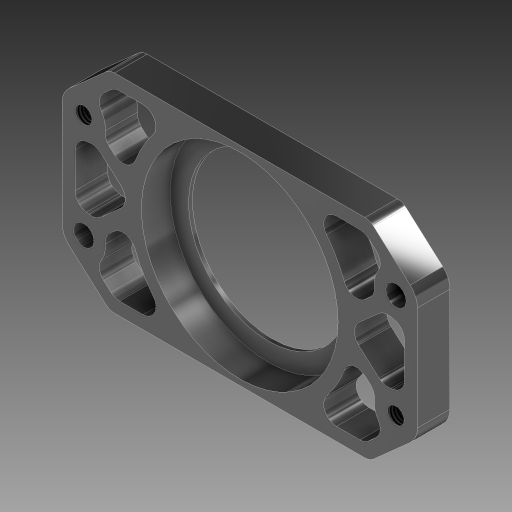
# Autodesk Inventor part: MaxSpline Bearing Block
Saved by Autodesk Inventor 2024 (Build 280153000, 153)
## iProperties
Created: 2023-05-20
Part Number: MaxSpline Bearing Block
Material: Aluminum 6061
Document SubType Name: Modeling
Designer: Max Boord
Mass: 47.5675 g
Surface Area: 134.115 cm^2
Volume: 17.6176 cm^3
Density: 2.7 g/cm^3
Appearance: Glazed - Black
Author: Max Boord
Mass: 32.2811 g
Surface Area: 98.3675 cm^2
Volume: 11.956 cm^3
Appearance: Aluminum - Flat
Autodesk Inventor part; units mm, degrees
ref_plane "YZ Plane" through (0, 0, 0) normal (1, 0, 0) x (0, 1, 0)
ref_plane "XZ Plane" through (0, 0, 0) normal (0, 1, 0) x (-1, 0, 0)
ref_plane "XY Plane" through (0, 0, 0) normal (0, 0, 1) x (1, 0, 0)
sketch "Sketch1" plane through (0, 0, 0) normal (0, 0, 1) x (1, 0, 0)
  circle A0 centre (0, 0) radius 24
  line L0 (31.75, 25.4) -> (-31.75, 25.4)
  line L1 (-31.75, 25.4) -> (-31.75, -25.4)
  line L2 (-31.75, -25.4) -> (31.75, -25.4)
  line L3 (31.75, -25.4) -> (31.75, 25.4)
  line L4 (31.75, 25.4) -> (-31.75, -25.4) construction
  line L5 (-31.75, 25.4) -> (31.75, -25.4) construction
  circle A1 centre (-38.1, 12.7) radius 2.4892 construction
  circle A2 centre (-38.1, -12.7) radius 2.4892
  circle A3 centre (38.1, 12.7) radius 2.4892
  circle A4 centre (38.1, -12.7) radius 2.4892 construction
  arc A5 (-41.6024, 16.6385) -> (-43.3705, 12.7) centre (-38.1, 12.7) ccw
  arc A6 (-43.3705, -12.7) -> (-41.6024, -16.6385) centre (-38.1, -12.7) ccw
  arc A7 (43.3705, 12.7) -> (41.6024, 16.6385) centre (38.1, 12.7) ccw
  arc A8 (41.6024, -16.6385) -> (43.3705, -12.7) centre (38.1, -12.7) ccw
  line L6 (-31.75, 25.4) -> (-41.6024, 16.6385)
  line L7 (-43.3705, 12.7) -> (-43.3705, -12.7)
  line L8 (-41.6024, -16.6385) -> (-31.75, -25.4)
  line L9 (31.75, 25.4) -> (41.6024, 16.6385)
  line L10 (43.3705, 12.7) -> (43.3705, -12.7)
  line L11 (41.6024, -16.6385) -> (31.75, -25.4)
  line L12 (-38.1, 12.7) -> (0, 0) construction
  line L13 (-38.1, -12.7) -> (0, 0) construction
  circle A9 centre (0, 0) radius 19.5
  circle A10 centre (-38.1, 12.7) radius 2.0193
  circle A11 centre (38.1, -12.7) radius 2.0193
  dimension "d0" = 48
  dimension "d1" = 50.8
  dimension "d2" = 4.9784
  dimension "d5" = 25.4
  dimension "d8" = 76.2
  dimension "d11" = 10.541
  dimension "d13" = 6.35
  dimension "d17" = 39
  dimension "d22" = 4.0386
  constraints: 28 end point, 12 centre point, 8 point on circle, 8 tangent, 4 equal radius, 2 coincident, 2 equal length, 2 horizontal, 2 midpoint, 2 parallel, 1 perpendicular, 1 vertical, 6 other
  measures "d0" diameter of A0
  measures "d1" distance of L1.end L0.end
  measures "d2" diameter of A1
  measures "d5" distance of L12.start L13.start
  measures "d8" distance of L12.start A3.centre
  measures "d11" diameter of A6
  measures "d13" distance from line of L1 L12.start
  measures "d17" diameter of A9
  measures "d22" diameter of A10
extrude "Extrusion1" add sketch "Sketch1" along normal blind 7 and the other way blind 0.9375 contours L3 L2 L1 L0 | L9 A7 L10 A8 L11 L3 | L1 L8 A6 L7 A5 L6
extrude "Extrusion2" add sketch "Sketch1" against normal up to surface (0.9375 mm away) contours A0
sketch "Sketch5" plane through (0, 0, 0) normal (0, 1, 0) x (-1, 0, 0)
  line L0 (-6.8199, 0) -> (-6.8199, 10.2616)
  line L1 (-24.003, 10.2616) -> (-24.003, 0)
  line L2 (-24.003, 0) -> (-6.8199, 10.2616) construction
  line L3 (-6.8199, 0) -> (-24.003, 10.2616) construction
  line L4 (-17.6085, 0) -> (-17.6085, 0.3048)
  line L5 (-17.6085, 0.3048) -> (-13.2143, 0.3048)
  line L6 (-13.2143, 0.3048) -> (-13.2143, 0)
  line L7 (-17.6086, 10.2616) -> (-17.6086, 9.9568)
  line L8 (-17.6086, 9.9568) -> (-13.2143, 9.9568)
  line L9 (-13.2143, 9.9568) -> (-13.2143, 10.2616)
  line L10 (-6.8199, 10.2616) -> (-13.2143, 10.2616)
  line L11 (-17.6086, 10.2616) -> (-24.003, 10.2616)
  line L12 (-24.003, 0) -> (-17.6085, 0)
  line L13 (-13.2143, 0) -> (-6.8199, 0)
  line L14 (0, 0) -> (0, -7.8157)
  line L15 (-24, 0) -> (24, 0) projected
  point P0 (-15.4115, 5.1308)
  dimension "d89" = 10.2616
  dimension "d90" = 13.6398
  dimension "d91" = 4.3942
  dimension "d92" = 0.3048
  dimension "d93" = 48.006
  constraints: 30 end point, 7 parallel, 6 equal length, 3 horizontal, 3 perpendicular, 2 midpoint, 1 collinear, 1 point on line, 1 vertical
  measures "d89" distance between parallel lines of L10 L13
  measures "d90" diameter of L0 L14
  measures "d91" distance of L7.end L8.end
  measures "d92" distance of L8.end L9.end
  measures "d93" diameter of L1 L14
revolve "Revolution1" [suppressed]
chamfer "Chamfer2" [suppressed]
sketch "Sketch2" plane through (0, 0, 7) normal (0, 0, 1) x (1, 0, 0)
  arc A0 (-41.6024, 16.6385) -> (-43.3705, 12.7) centre (-38.1, 12.7) ccw projected
  line L0 (-43.3705, 12.7) -> (-43.3705, -12.7) projected
  arc A1 (-43.3705, -12.7) -> (-41.6024, -16.6385) centre (-38.1, -12.7) ccw projected
  line L1 (-41.6024, -16.6385) -> (-31.75, -25.4) projected
  line L2 (-31.75, -25.4) -> (31.75, -25.4) projected
  line L3 (31.75, -25.4) -> (41.6024, -16.6385) projected
  arc A2 (41.6024, -16.6385) -> (43.3705, -12.7) centre (38.1, -12.7) ccw projected
  line L4 (43.3705, -12.7) -> (43.3705, 12.7) projected
  arc A3 (43.3705, 12.7) -> (41.6024, 16.6385) centre (38.1, 12.7) ccw projected
  line L5 (41.6024, 16.6385) -> (31.75, 25.4) projected
  line L6 (31.75, 25.4) -> (-31.75, 25.4) projected
  line L7 (-31.75, 25.4) -> (-41.6024, 16.6385) projected
  circle A4 centre (38.1, -12.7) radius 2.0193 projected
  circle A5 centre (38.1, 12.7) radius 2.4892 projected
  circle A6 centre (0, 0) radius 24 projected
  circle A7 centre (-38.1, -12.7) radius 2.4892 projected
  circle A8 centre (-38.1, 12.7) radius 2.0193 projected
  line L8 (30.5425, -22.225) -> (-30.5425, -22.225)
  line L9 (-30.5425, -22.225) -> (-39.4925, -14.2659)
  arc A9 (-40.1955, -12.7) -> (-39.4925, -14.2659) centre (-38.1, -12.7) ccw
  line L10 (-40.1955, -12.7) -> (-40.1955, 12.7)
  arc A10 (-39.4925, 14.2659) -> (-40.1955, 12.7) centre (-38.1, 12.7) ccw
  line L11 (-39.4925, 14.2659) -> (-30.5425, 22.225)
  line L12 (-30.5425, 22.225) -> (30.5425, 22.225)
  line L13 (30.5425, 22.225) -> (39.4925, 14.2659)
  arc A11 (40.1955, 12.7) -> (39.4925, 14.2659) centre (38.1, 12.7) ccw
  line L14 (40.1955, 12.7) -> (40.1955, -12.7)
  arc A12 (39.4925, -14.2659) -> (40.1955, -12.7) centre (38.1, -12.7) ccw
  line L15 (39.4925, -14.2659) -> (30.5425, -22.225)
  circle A13 centre (0, 0) radius 27.175
  circle A14 centre (38.1, -12.7) radius 5.2705
  circle A15 centre (38.1, 12.7) radius 5.2705
  circle A16 centre (-38.1, 12.7) radius 5.2705
  circle A17 centre (-38.1, -12.7) radius 5.2705
  line L16 (38.1, -12.7) -> (24, 0) construction
  line L17 (39.1624, -11.5204) -> (25.0624, 1.1796)
  line L18 (22.9376, -1.1796) -> (37.0376, -13.8796)
  arc A18 (37.0376, -13.8796) -> (39.1624, -11.5204) centre (38.1, -12.7) ccw
  arc A19 (25.0624, 1.1796) -> (22.9376, -1.1796) centre (24, 0) ccw
  line L19 (24, 0) -> (38.1, 12.7) construction
  line L20 (25.0624, -1.1796) -> (39.1624, 11.5204)
  line L21 (37.0376, 13.8796) -> (22.9376, 1.1796)
  arc A20 (22.9376, 1.1796) -> (25.0624, -1.1796) centre (24, 0) ccw
  arc A21 (39.1624, 11.5204) -> (37.0376, 13.8796) centre (38.1, 12.7) ccw
  line L22 (0, 0) -> (0, -25.4)
  line L23 (-39.1624, -11.5204) -> (-25.0624, 1.1796)
  line L24 (-22.9376, -1.1796) -> (-37.0376, -13.8796)
  line L25 (-25.0624, -1.1796) -> (-39.1624, 11.5204)
  line L26 (-37.0376, 13.8796) -> (-22.9376, 1.1796)
  point P0 (31.05, -6.35)
  point P1 (31.05, 6.35)
  point P2 (26.7764, 4.6373)
  point P3 (33.3033, 10.5161)
  point P4 (35.8787, 17.4796)
  point P5 (15.6375, 22.225)
  point P6 (35.4282, 8.1569)
  point P7 (27.1656, 0.7148)
  point P8 (27.1656, -0.7148)
  point P9 (35.4282, -8.1569)
  point P10 (40.1955, -7.864)
  point P11 (40.1955, 7.864)
  point P12 (33.3033, -10.5161)
  point P13 (26.7764, -4.6373)
  point P14 (15.6375, -22.225)
  point P15 (35.8787, -17.4796)
  point P16 (-26.7764, -4.6373)
  point P17 (-33.3033, -10.5161)
  point P18 (-35.8787, -17.4796)
  point P19 (-15.6375, -22.225)
  point P20 (-27.1656, 0.7148)
  point P21 (-35.4282, 8.1569)
  point P22 (-40.1955, 7.864)
  point P23 (-40.1955, -7.864)
  point P24 (-35.4282, -8.1569)
  point P25 (-27.1656, -0.7148)
  point P26 (-33.3033, 10.5161)
  point P27 (-26.7764, 4.6373)
  point P28 (-15.6375, 22.225)
  point P29 (-35.8787, 17.4796)
  dimension "d23" = 3.175
  dimension "d24" = 3.175
  dimension "d25" = 3.175
  dimension "d26" = 3.175
  constraints: 42 end point, 16 point on circle, 10 centre point, 8 symmetric about line, 8 tangent, 4 coincident, 3 midpoint, 2 parallel, 1 equal length, 1 horizontal alignment, 22 other
  measures "d23" distance between parallel lines of L2 L8
  measures "d25" diameter of A19
  measures "d26" diameter of A21
extrude "Extrusion3" cut sketch "Sketch2" against normal through all contours L11 L12 A13 L26 A16 | A16 L25 A13 L23 A17 L10 | A17 L24 A13 L8 L9 | L12 L13 A15 L21 A13 | L20 A15 L14 A14 L17 A13 | A13 L18 A14 L15 L8
fillet "Fillet1" radius 3.175 36 edges at (-26.7764, -4.6373, 3.0313) (-33.3033, -10.5161, 3.0313) (-35.8787, -17.4796, 3.0313) (-30.5425, -22.225, 3.0313) (-15.6375, -22.225, 3.0313) (26.7764, 4.6373, 3.0313) (33.3033, 10.5161, 3.0313) (35.8787, 17.4796, 3.0313) (30.5425, 22.225, 3.0313) (15.6375, 22.225, 3.0313) (-27.1656, -0.7148, 3.0313) (-27.1656, 0.7148, 3.0313) (-35.4282, 8.1569, 3.0313) (-40.1955, 7.864, 3.0313) (-40.1955, -7.864, 3.0313) (-35.4282, -8.1569, 3.0313) (33.3033, -10.5161, 3.0313) (26.7764, -4.6373, 3.0313) (15.6375, -22.225, 3.0313) (30.5425, -22.225, 3.0313) (35.8787, -17.4796, 3.0313) (40.1955, 7.864, 3.0313) (35.4282, 8.1569, 3.0313) (27.1656, 0.7148, 3.0313) (27.1656, -0.7148, 3.0313) (35.4282, -8.1569, 3.0313) (40.1955, -7.864, 3.0313) (-33.3033, 10.5161, 3.0313) (-26.7764, 4.6373, 3.0313) (-15.6375, 22.225, 3.0313) (-30.5425, 22.225, 3.0313) (-35.8787, 17.4796, 3.0313) (31.75, 25.4, 3.0313) (-31.75, 25.4, 3.0313) (31.75, -25.4, 3.0313) (-31.75, -25.4, 3.0313)
thread "Thread1" size "10-32 UNF" class "2B" standard "ANSI Unified Screw Threads" length 12.7
thread "Thread2" size "10-32 UNF" class "2B" standard "ANSI Unified Screw Threads" length 12.7
delete_face "Delete Face1" [suppressed]
sketch "Sketch3" plane through (-43.3705, -12.7, 7) normal (0, 0, 1) x (1, 0, 0)
  arc A0 (73.913, -12.7) -> (76.0228, -11.8976) centre (73.913, -9.525) ccw projected
  line L0 (76.0228, -11.8976) -> (84.9729, -3.9385) projected
  arc A1 (84.9729, -3.9385) -> (86.741, 0) centre (81.4705, 0) ccw projected
  line L1 (86.741, 0) -> (86.741, 25.4) projected
  arc A2 (86.741, 25.4) -> (84.9729, 29.3385) centre (81.4705, 25.4) ccw projected
  line L2 (84.9729, 29.3385) -> (76.0228, 37.2976) projected
  arc A3 (76.0228, 37.2976) -> (73.913, 38.1) centre (73.913, 34.925) ccw projected
  line L3 (73.913, 38.1) -> (12.828, 38.1) projected
  arc A4 (12.828, 38.1) -> (10.7182, 37.2976) centre (12.828, 34.925) ccw projected
  line L4 (10.7182, 37.2976) -> (1.7681, 29.3385) projected
  arc A5 (1.7681, 29.3385) -> (0, 25.4) centre (5.2705, 25.4) ccw projected
  line L5 (0, 25.4) -> (0, 0) projected
  arc A6 (0, 0) -> (1.7681, -3.9385) centre (5.2705, 0) ccw projected
  line L6 (1.7681, -3.9385) -> (10.7182, -11.8976) projected
  arc A7 (10.7182, -11.8976) -> (12.828, -12.7) centre (12.828, -9.525) ccw projected
  line L7 (12.828, -12.7) -> (73.913, -12.7) projected
  circle A8 centre (81.4705, 0) radius 2.0193 projected
  circle A9 centre (81.4705, 25.4) radius 2.4892 projected
  circle A10 centre (43.3705, 12.7) radius 24 projected
  circle A11 centre (81.4705, 25.4) radius 2.4892
  circle A12 centre (81.4705, 0) radius 2.4892
  circle A13 centre (68.7705, 25.4) radius 2.4892
  circle A14 centre (68.7705, 0) radius 2.4892
  circle A15 centre (56.0705, 25.4) radius 2.4892
  circle A16 centre (56.0705, 0) radius 2.4892
  circle A17 centre (43.3705, 25.4) radius 2.4892
  circle A18 centre (43.3705, 0) radius 2.4892
  dimension "d48" = 25.4
  dimension "d51" = 12.7
  constraints: 8 centre point, 1 coincident, 1 concentric, 1 horizontal, 1 vertical, 14 other
  measures "d48" distance of A11.centre A12.centre
  measures "d51" distance of A11.centre A13.centre
extrude "Extrusion4" [suppressed]
sketch "Sketch4" plane through (-43.3705, -12.7, 7) normal (0, 0, 1) x (1, 0, 0)
  arc A0 (73.913, -12.7) -> (76.0228, -11.8976) centre (73.913, -9.525) ccw projected
  line L0 (76.0228, -11.8976) -> (84.9729, -3.9385) projected
  arc A1 (84.9729, -3.9385) -> (86.741, 0) centre (81.4705, 0) ccw projected
  line L1 (86.741, 0) -> (86.741, 25.4) projected
  arc A2 (86.741, 25.4) -> (84.9729, 29.3385) centre (81.4705, 25.4) ccw projected
  line L2 (84.9729, 29.3385) -> (76.0228, 37.2976) projected
  arc A3 (76.0228, 37.2976) -> (73.913, 38.1) centre (73.913, 34.925) ccw projected
  line L3 (73.913, 38.1) -> (12.828, 38.1) projected
  arc A4 (12.828, 38.1) -> (10.7182, 37.2976) centre (12.828, 34.925) ccw projected
  line L4 (10.7182, 37.2976) -> (1.7681, 29.3385) projected
  arc A5 (1.7681, 29.3385) -> (0, 25.4) centre (5.2705, 25.4) ccw projected
  line L5 (0, 25.4) -> (0, 0) projected
  arc A6 (0, 0) -> (1.7681, -3.9385) centre (5.2705, 0) ccw projected
  line L6 (1.7681, -3.9385) -> (10.7182, -11.8976) projected
  arc A7 (10.7182, -11.8976) -> (12.828, -12.7) centre (12.828, -9.525) ccw projected
  line L7 (12.828, -12.7) -> (73.913, -12.7) projected
  circle A8 centre (81.4705, 25.4) radius 2.4892 projected
  circle A9 centre (43.3705, 12.7) radius 24 projected
  line L8 (73.913, -9.525) -> (82.863, -1.5659)
  arc A10 (82.863, -1.5659) -> (83.566, 0) centre (81.4705, 0) ccw
  line L9 (83.566, 0) -> (83.566, 25.4)
  arc A11 (83.566, 25.4) -> (82.863, 26.9659) centre (81.4705, 25.4) ccw
  line L10 (82.863, 26.9659) -> (73.913, 34.925)
  line L11 (73.913, 34.925) -> (12.828, 34.925)
  line L12 (12.828, 34.925) -> (3.878, 26.9659)
  arc A12 (3.878, 26.9659) -> (3.175, 25.4) centre (5.2705, 25.4) ccw
  line L13 (3.175, 25.4) -> (3.175, 0)
  arc A13 (3.175, 0) -> (3.878, -1.5659) centre (5.2705, 0) ccw
  line L14 (3.878, -1.5659) -> (12.828, -9.525)
  line L15 (12.828, -9.525) -> (73.913, -9.525)
  circle A14 centre (43.3705, 12.7) radius 27.175
  circle A15 centre (85.3694, 0) radius 4.2164
  circle A16 centre (72.6694, 0) radius 4.2164
  circle A17 centre (59.9694, 0) radius 4.2164
  circle A18 centre (47.2694, 0) radius 4.2164
  circle A19 centre (85.3694, 25.4) radius 4.2164
  circle A20 centre (72.6694, 25.4) radius 4.2164
  circle A21 centre (59.9694, 25.4) radius 4.2164
  circle A22 centre (47.2694, 25.4) radius 4.2164
  line L16 (85.3694, 0) -> (47.2694, 0) construction
  line L17 (85.3694, 3.175) -> (47.2694, 3.175)
  line L18 (47.2694, -3.175) -> (85.3694, -3.175)
  arc A23 (85.3694, -3.175) -> (85.3694, 3.175) centre (85.3694, 0) ccw
  arc A24 (47.2694, 3.175) -> (47.2694, -3.175) centre (47.2694, 0) ccw
  line L19 (85.3694, 25.4) -> (47.2694, 25.4) construction
  line L20 (85.3694, 28.575) -> (47.2694, 28.575)
  line L21 (47.2694, 22.225) -> (85.3694, 22.225)
  arc A25 (85.3694, 22.225) -> (85.3694, 28.575) centre (85.3694, 25.4) ccw
  arc A26 (47.2694, 28.575) -> (47.2694, 22.225) centre (47.2694, 25.4) ccw
  line L22 (59.9694, 0) -> (59.9694, -12.7) construction
  line L23 (58.3819, 0) -> (58.3819, -12.7)
  line L24 (61.5569, -12.7) -> (61.5569, 0)
  arc A27 (61.5569, 0) -> (58.3819, 0) centre (59.9694, 0) ccw
  arc A28 (58.3819, -12.7) -> (61.5569, -12.7) centre (59.9694, -12.7) ccw
  line L25 (59.9694, 25.4) -> (59.9694, 38.1) construction
  line L26 (61.5569, 25.4) -> (61.5569, 38.1)
  line L27 (58.3819, 38.1) -> (58.3819, 25.4)
  arc A29 (58.3819, 25.4) -> (61.5569, 25.4) centre (59.9694, 25.4) ccw
  arc A30 (61.5569, 38.1) -> (58.3819, 38.1) centre (59.9694, 38.1) ccw
  line L28 (85.3694, 0) -> (94.358, 12.7) construction
  line L29 (86.6652, -0.9171) -> (95.6538, 11.7829)
  line L30 (93.0622, 13.6171) -> (84.0736, 0.9171)
  arc A31 (84.0736, 0.9171) -> (86.6652, -0.9171) centre (85.3694, 0) ccw
  arc A32 (95.6538, 11.7829) -> (93.0622, 13.6171) centre (94.358, 12.7) ccw
  line L31 (94.358, 12.7) -> (85.3694, 25.4) construction
  line L32 (95.6538, 13.6171) -> (86.6652, 26.3171)
  line L33 (84.0736, 24.4829) -> (93.0622, 11.7829)
  arc A33 (93.0622, 11.7829) -> (95.6538, 13.6171) centre (94.358, 12.7) ccw
  arc A34 (86.6652, 26.3171) -> (84.0736, 24.4829) centre (85.3694, 25.4) ccw
  line L34 (73.9652, -0.9171) -> (82.9538, 11.7829)
  line L35 (80.3622, 13.6171) -> (71.3736, 0.9171)
  line L36 (71.3736, 24.4829) -> (80.3622, 11.7829)
  line L37 (82.9538, 13.6171) -> (73.9652, 26.3171)
  arc A35 (80.3622, 11.7829) -> (82.9538, 13.6171) centre (81.658, 12.7) ccw
  arc A36 (82.9538, 11.7829) -> (80.3622, 13.6171) centre (81.658, 12.7) ccw
  line L38 (61.2652, -0.9171) -> (70.2538, 11.7829)
  line L39 (67.6622, 13.6171) -> (58.6736, 0.9171)
  line L40 (58.6736, 24.4829) -> (67.6622, 11.7829)
  line L41 (70.2538, 13.6171) -> (61.2652, 26.3171)
  arc A37 (67.6622, 11.7829) -> (70.2538, 13.6171) centre (68.958, 12.7) ccw
  arc A38 (70.2538, 11.7829) -> (67.6622, 13.6171) centre (68.958, 12.7) ccw
  line L42 (68.958, 12.7) -> (86.741, 12.7) construction
  line L43 (66.1704, 11.5094) -> (86.741, 11.5094)
  line L44 (86.741, 13.8906) -> (66.1704, 13.8906)
  arc A39 (68.958, 13.8906) -> (68.958, 11.5094) centre (68.958, 12.7) ccw
  arc A40 (86.741, 11.5094) -> (86.741, 13.8906) centre (86.741, 12.7) ccw
  circle A41 centre (85.3694, 0) radius 2.4892
  circle A42 centre (85.3694, 25.4) radius 2.4892
  circle A43 centre (76.6953, 0) radius 2.4892 projected
  point P0 (66.3194, 0)
  point P1 (66.3194, 25.4)
  point P2 (59.9694, -6.35)
  point P3 (59.9694, 31.75)
  point P4 (89.8637, 6.35)
  point P5 (89.8637, 19.05)
  point P6 (77.8495, 12.7)
  point P7 (61.5569, 34.925)
  point P8 (61.5569, 29.3061)
  point P9 (62.7438, 28.575)
  point P10 (69.895, 28.575)
  point P11 (75.4438, 28.575)
  point P12 (82.595, 28.575)
  point P13 (81.9112, 27.8123)
  point P14 (58.3819, 29.3061)
  point P15 (58.3819, 34.925)
  point P16 (59.008, 34.925)
  point P17 (50.7411, 30.1301)
  point P18 (50.0438, 28.575)
  point P19 (57.195, 28.575)
  point P20 (70.0602, 13.8906)
  point P21 (78.8704, 13.8906)
  point P22 (72.9717, 22.225)
  point P23 (62.7438, 22.225)
  point P24 (63.5218, 23.1288)
  point P25 (82.7602, 13.8906)
  point P26 (78.9628, 13.8906)
  point P27 (91.6608, 22.225)
  point P28 (75.4438, 22.225)
  point P29 (76.2218, 23.1288)
  point P30 (82.9036, 13.8906)
  point P31 (83.566, 13.8906)
  point P32 (83.566, 21.5887)
  point P33 (88.9218, 23.1288)
  point P34 (83.566, 11.5094)
  point P35 (82.9036, 11.5094)
  point P36 (88.9218, 2.2712)
  point P37 (83.566, 3.8113)
  point P38 (78.8704, 11.5094)
  point P39 (70.0602, 11.5094)
  point P40 (63.5218, 2.2712)
  point P41 (62.7438, 3.175)
  point P42 (72.9717, 3.175)
  point P43 (78.9628, 11.5094)
  point P44 (82.7602, 11.5094)
  point P45 (76.2218, 2.2712)
  point P46 (75.4438, 3.175)
  point P47 (91.6608, 3.175)
  point P48 (61.5569, -3.9061)
  point P49 (61.5569, -9.525)
  point P50 (81.9112, -2.4123)
  point P51 (82.595, -3.175)
  point P52 (75.4438, -3.175)
  point P53 (69.895, -3.175)
  point P54 (62.7438, -3.175)
  point P55 (58.3819, -9.525)
  point P56 (58.3819, -3.9061)
  point P57 (57.195, -3.175)
  point P58 (50.0438, -3.175)
  point P59 (50.7411, -4.7301)
  point P60 (59.008, -9.525)
  point P61 (55.9243, 17.1025)
  point P62 (60.2717, 22.225)
  point P63 (50.0438, 22.225)
  point P64 (54.7469, 22.1185)
  point P65 (60.2717, 3.175)
  point P66 (55.9243, 8.2975)
  point P67 (54.7469, 3.2815)
  point P68 (50.0438, 3.175)
  point P69 (70.008, 11.5094)
  point P70 (53.3788, 11.7596)
  point P71 (60.9302, 4.1055)
  point P72 (60.9302, 21.2945)
  point P73 (53.3788, 13.6404)
  point P74 (70.008, 13.8906)
  point P75 (57.195, 3.175)
  point P76 (57.195, 22.225)
  point P77 (70.5194, 11.5094)
  point P78 (70.5194, 13.8906)
  point P79 (82.595, 22.225)
  point P80 (58.3819, 28.575)
  point P81 (81.3178, 28.34)
  point P82 (81.0536, 28.575)
  point P83 (61.5569, 28.575)
  point P84 (76.708, 32.4394)
  point P85 (79.883, 29.616)
  point P86 (83.566, 22.225)
  point P87 (80.8624, 28.745)
  point P88 (27.733, -9.525)
  point P89 (27.733, 34.925)
  point P90 (68.8215, 22.225)
  point P91 (53.7027, 24.8603)
  point P92 (82.708, 11.5094)
  point P93 (103.3315, 22.225)
  point P94 (73.6302, 21.2945)
  point P95 (69.895, 22.225)
  point P96 (80.608, 11.5094)
  point P97 (76.8614, 22.225)
  point P98 (86.3302, 21.2945)
  point P99 (86.3302, 4.1055)
  point P100 (82.708, 13.8906)
  point P101 (103.3315, 3.175)
  point P102 (73.6302, 4.1055)
  point P103 (80.608, 13.8906)
  point P104 (69.895, 3.175)
  point P105 (76.8614, 3.175)
  point P106 (82.595, 3.175)
  point P107 (61.5569, -3.175)
  point P108 (81.0536, -3.175)
  point P109 (81.3178, -2.94)
  point P110 (58.3819, -3.175)
  point P111 (83.566, 3.175)
  point P112 (79.883, -4.216)
  point P113 (76.708, -7.0394)
  point P114 (80.8624, -3.345)
  point P115 (68.8215, 3.175)
  point P116 (53.7027, 0.5397)
  point P117 (56.2407, 13.227)
  point P118 (64.1614, 3.175)
  point P119 (56.2407, 12.173)
  point P120 (64.1614, 22.225)
  point P121 (65.4265, -3.175)
  point P122 (65.4265, 28.575)
  point P123 (63.9953, 23.8125)
  point P124 (63.9953, 1.5875)
  point P125 (89.3953, -1.5875)
  point P126 (88.2537, 1.3273)
  point P127 (89.3953, -1.5875)
  point P128 (89.3953, 26.9875)
  point P129 (88.2537, 24.0727)
  point P130 (89.3953, 26.9875)
  dimension "d56" = 3.175
  dimension "d57" = 3.175
  dimension "d58" = 8.4328
  dimension "d61" = 12.7
  dimension "d64" = 25.4
  dimension "d67" = 6.35
  dimension "d68" = 3.175
  dimension "d69" = 3.175
  dimension "d70" = 3.175
  dimension "d71" = 3.175
  dimension "d74" = 12.7
  dimension "d79" = 2.3813
  dimension "d88" = 1.3716
  constraints: 88 end point, 44 point on circle, 33 centre point, 29 tangent, 8 midpoint, 7 parallel, 7 point on line, 5 horizontal, 3 equal radius, 2 coincident, 1 equal length, 1 perpendicular, 1 vertical, 55 other
  measures "d56" distance between parallel lines of L7 L15
  measures "d57" radial gap between concentric circles of A9 A14
  measures "d58" diameter of A15
  measures "d61" distance of L16.start A16.centre
  measures "d64" distance of L16.start L19.start
  measures "d67" diameter of A24
  measures "d68" diameter of A28
  measures "d69" diameter of A30
  measures "d70" diameter of A32
  measures "d71" diameter of A34
  measures "d74" distance of L29.start L34.start
  measures "d79" diameter of A40
  measures "d88" distance from line of L1 A41.centre
extrude "Extrusion5" [suppressed]
fillet "Fillet2" [suppressed]
fillet "Fillet3" [suppressed]
chamfer "Chamfer1" [suppressed]
body "Solid1"
body "Solid2"
